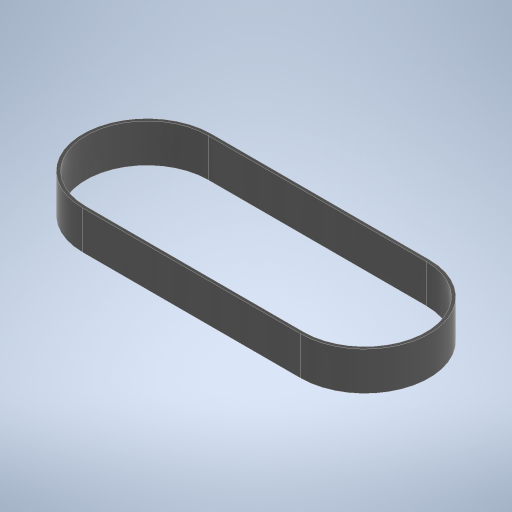
# Autodesk Inventor part: 2309HCMUTE-CDT23-BELT_S5M-320X64X15
Saved by Autodesk Inventor 2023 (Build 270158000, 158)
## iProperties
Created: 2023-11-01
Part Number: 2309HCMUTE-CDT23-BELT_S5M-320X64X15
Material: Rubber
Document SubType Name: Modeling
Designer: havie
Density: 0.93 g/cm^3
Appearance: Dark Gray
Author: havie
Autodesk Inventor part; units mm, degrees
ref_plane "YZ Plane" through (0, 0, 0) normal (1, 0, 0) x (0, 1, 0)
ref_plane "XZ Plane" through (0, 0, 0) normal (0, 1, 0) x (-1, 0, 0)
sketch "Sketch1" plane through (0, 0, 0) normal (0, 1, 0) x (-1, 0, 0)
  line L0 (42.5, 0) -> (-42.5, 0) construction
  line L1 (42.5, 23.8855) -> (-42.5, 23.8855)
  line L2 (-42.5, -23.8855) -> (42.5, -23.8855)
  arc A0 (42.5, -23.8855) -> (42.5, 23.8855) centre (42.5, 0) ccw
  arc A1 (-42.5, 23.8855) -> (-42.5, -23.8855) centre (-42.5, 0) ccw
  point P0 (0, 0)
  point P1 (0, 0)
  dimension "d0" = 85
  dimension "d1" = 47.771
  constraints: 8 end point, 4 point on circle, 4 tangent, 2 centre point, 1 coincident, 1 horizontal, 1 midpoint, 1 parallel
  measures "d0" distance of L1.start L1.end
  measures "d1" distance between parallel lines of L2 L1
ref_plane "Work Plane1" through (-42.5, 0, -23.8855) normal (-1, 0, 0) x (0, -1, 0)
sketch "Sketch2" plane through (-42.5, 0, -23.8855) normal (-1, 0, 0) x (0, -1, 0)
  line L0 (7.5, 0) -> (-7.5, 0)
  line L1 (-7.5, 0) -> (-7.5, -1.2)
  line L2 (-7.5, -1.2) -> (7.5, -1.2)
  line L3 (7.5, -1.2) -> (7.5, 0)
  line L4 (7.5, 0) -> (-7.5, -1.2) construction
  line L5 (-7.5, 0) -> (7.5, -1.2) construction
  point P0 (0, 23.8855)
  point P1 (0, -0.6)
  point P2 (0, 0)
  dimension "d2" = 15
  dimension "d3" = 1.2
  constraints: 10 end point, 2 midpoint, 2 parallel, 1 horizontal, 1 perpendicular, 4 other
  measures "d2" distance of L1.end L2.end
  measures "d3" distance of L2.end L0.start
sweep "Sweep1" add profiles "Sketch2" path "Sketch1"
body "Solid1"
